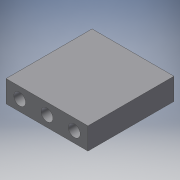
# Autodesk Inventor part: cycloid_base_bottom
Saved by Autodesk Inventor 2019.4 (Build 234330000, 330)
## iProperties
Created: 2019-08-28
Part Number: cycloid_base_bottom
Material: Generic
Document SubType Name: Modeling
Designer: cdi
Density: 1 g/cm^3
Appearance: Default
Author: cdi
Autodesk Inventor part; units mm, degrees
ref_plane "YZ Plane" through (0, 0, 0) normal (1, 0, 0) x (0, 1, 0)
ref_plane "XZ Plane" through (0, 0, 0) normal (0, 1, 0) x (-1, 0, 0)
ref_plane "XY Plane" through (0, 0, 0) normal (0, 0, 1) x (1, 0, 0)
sketch "Sketch1" plane through (0, 0, 0) normal (0, 0, 1) x (1, 0, 0)
  line L0 (-15, -4) -> (15, -4)
  line L1 (15, -4) -> (15, 4)
  line L2 (15, 4) -> (-15, 4)
  line L3 (-15, 4) -> (-15, -4)
  line L4 (-15, -4) -> (15, 4) construction
  line L5 (15, -4) -> (-15, 4) construction
  point P0 (0, 0)
  dimension "d0" = 8
  dimension "d1" = 30
  constraints: 12 end point, 2 midpoint, 2 parallel, 1 horizontal, 1 perpendicular
  measures "d0" distance of L0.end L1.end
  measures "d1" distance of L1.end L2.end
extrude "Extrusion1" add sketch "Sketch1" along normal blind 15.75 and the other way blind 15.75
sketch "Sketch2" plane through (0, 0, 15.75) normal (0, 0, 1) x (1, 0, 0)
  circle A0 centre (0, 0) radius 1.5
  dimension "d4" = 3
  constraints: 1 centre point, 1 coincident
  measures "d4" diameter of A0
hole "Hole1" at (0, 0, 15.75) direction (0, 0, -1) diameter 3.88 depth 7 countersink diameter 4.34 countersink angle 7
pattern_linear "Rectangular Pattern1" count 2 spacing 10 along (-1, 0, 0) count 2 spacing 10 along (1, 0, 0) of "Hole1"
mirror "Mirror1" about plane through (0, 0, 0) normal (0, 0, 1) of "Hole1", "Rectangular Pattern1"
body "Solid1"
